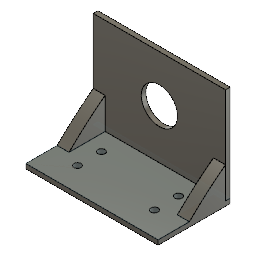
Motor Clamp v1 (Autodesk Fusion 360 design; units mm, degrees)
Autodesk Fusion 360 part; units mm, degrees
note: some values were not read from the file. Chosen so that the rebuilt part matches the saved one: which face or edge a step refers to; which pieces of a blend or face edit are solid.
box "BoxPrimitive1" add length 30 width 55 height 2 placed x (0, 0, 1) y (1, 0, 0) z (0, 1, 0) at (-30, 0, -20) makes body 1
box "BoxPrimitive2" add length 40 width 55 height 2 placed x (0, 1, 0) y (-1, 0, 0) z (0, 0, 1) at (44.5, 16.6, 0) separate body makes body 2
move_body "Move1" bodies 2 to x (1, 0, 0) y (0, 1, 0) z (0, 0, 1) at (-19.4581, -14.5906, -19.9832)
move_body "Move2" bodies 2 to x (1, 0, 0) y (0, 1, 0) z (0, 0, 1) at (-0.038, -0.0121, -0.0185)
sketch "Sketch7" plane through (0, 0, 0) normal (1, 0, 0) x (0, 0, -1)
sketch "Sketch8" plane through (0, 0, 0) normal (0, 0, 1) x (1, 0, 0)
  line L0 (-30, 15) -> (-25, 15)
  line L1 (-25, 15) -> (-25, 2)
  line L2 (-25, 2) -> (-30, 2)
  line L3 (-30, 2) -> (-30, 15)
  constraint horizontal L0
  constraint vertical L1
  constraint horizontal L2
  constraint vertical L3
extrude "Extrude1" add sketch "Sketch8" against normal blind 18 bodies 1
extrude "Extrude2" cut 1 faces at (-28.3333, 10.6667, 0) along direction (0, 0, -1) blind 3 on bodies 1 bodies 1
sketch "Sketch9" plane through (0, 0, -3) normal (0, 0, 1) x (1, 0, 0)
  line L0 (-30, 2) -> (-25, 2)
  line L1 (-25, 2) -> (-25, 15)
  line L2 (-25, 15) -> (-30, 15)
  line L3 (-30, 15) -> (-30, 2)
  line L4 (25, 15) -> (20, 15)
  line L5 (20, 15) -> (20, 2)
  line L6 (20, 2) -> (25, 2)
  line L7 (25, 2) -> (25, 15)
  constraint horizontal L4
  constraint vertical L5
  constraint horizontal L6
  constraint vertical L7
extrude "Extrude3" add sketch "Sketch9" against normal blind 15 contours L4 L5 L6 L7 bodies 1
chamfer "Chamfer1" distance 13 angle 45 1 edges at (-27.5, 15, -3) on bodies 1
fillet "Fillet1" radius 146 1 edges at (-27.5, 15, -16) on bodies 1
chamfer "Chamfer2" distance 13 angle 45 1 edges at (22.5, 15, -3) on bodies 1
fillet "Fillet2" radius 140 1 edges at (22.5, 15, -16) on bodies 1
hole "Hole1" at (-2.4961, 21.9973, -18.0017) direction (0, 0, -1) diameter 15 depth 17 tip angle 118 bodies 2
move_face "MoveFace1" to x (1, 0, 0) y (0, 1, 0) z (0, 0, 1) at (0, 0.5, 0) 1 faces at (-1.7494, 14.5346, -19.335) on bodies 2
sketch "Sketch10" plane through (0, 2, 0) normal (0, 1, 0) x (-1, 0, 0)
  line L0 (-25, -3) -> (-20, -3)
  line L1 (-20, -3) -> (-20, -18)
  line L2 (-20, -18) -> (-25, -18)
  line L3 (-25, -18) -> (-25, -20)
  line L4 (-25, -20) -> (30, -20)
  line L5 (30, -20) -> (30, -18)
  line L6 (30, -18) -> (25, -18)
  line L7 (25, -18) -> (25, -3)
  line L8 (25, -3) -> (30, -3)
  line L9 (30, -3) -> (30, 10)
  line L10 (30, 10) -> (-25, 10)
  line L11 (-25, 10) -> (-25, -3)
hole "Hole4" at (-18.4996, 2, -9.9999) direction (0, -1, 0) diameter 3 depth 3 tip angle 118 bodies 1
hole "Hole2" at (13.5, 2, 0.0001) direction (0, -1, 0) diameter 3 depth 3 tip angle 118 bodies 1
hole "Hole3" at (-18.5, 2, -0.0002) direction (0, -1, 0) diameter 3 depth 3 tip angle 118 bodies 1
hole "Hole5" at (13.5, 2, -9.9998) direction (0, -1, 0) diameter 3 depth 3 tip angle 118 bodies 1
sketch "Sketch11" plane through (0, 0, 0) normal (1, 0, 0) x (0, 0, -1)
sketch "Sketch12" plane through (0, 0, 0) normal (1, 0, 0) x (0, 0, -1)
combine "Combine1" operation add target body 1 tool bodies 2
